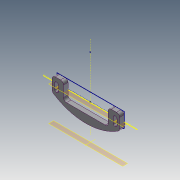
# Autodesk Inventor part: J005684
Saved by Autodesk Inventor 2015 SP1 (Build 190203100, 203)
## iProperties
Created: 2014-12-01
Material: Generic
Vendor: HHMI: JFRC - ID&F
Document SubType Name: Modeling
Designer: ARNOLDJ
Density: 1 g/cm^3
Appearance: Default
Part Number: J005684
Description: SIDE BALL GUIDE
RuleStatus: InUse
AfterDocSave0: file://Part Number Cleaner
DESIGN DEPARTMENT: HHMI: JFRC - ID&F
ALTERED ITEM PART NUMBER: N/A
ALTERED ITEM VENDOR: N/A
ALTERED ITEM DESCRIPTION: N/A
Author: ARNOLDJ
Revision Number: 0
Autodesk Inventor part; units mm, degrees
sketch "Sketch1" plane through (0, 0, 0) normal (0, 0, 1) x (1, 0, 0)
  line L0 (-100.457, 0) -> (100.457, 0) construction
  line L1 (0, 116.967) -> (0, -60.833) construction
  circle A0 centre (-62.4459, 0) radius 3.8354 construction
  circle A1 centre (62.4459, 0) radius 3.8354 construction
  line L2 (-62.4459, 0) -> (62.4459, 0) construction
  line L3 (-71.755, 17.78) -> (71.755, 17.78)
  line L4 (71.755, 17.78) -> (71.755, -13.2195)
  line L5 (-71.755, -13.2195) -> (-71.755, 17.78)
  circle A2 centre (-64.3509, 0) radius 3.8354 construction
  circle A3 centre (-60.5409, 0) radius 3.8354 construction
  line L6 (-64.3559, 3.8354) -> (-60.5409, 3.8354) construction
  line L7 (-64.3763, -3.8353) -> (-60.541, -3.8354) construction
  circle A4 centre (62.4459, 0) radius 3.8354 construction
  arc A5 (-71.755, -13.2195) -> (71.755, -13.2195) centre (0, 91.567) ccw
  line L8 (66.2813, -9.525) -> (58.6105, -9.525)
  line L9 (58.6105, -9.525) -> (58.6105, 9.525)
  line L10 (58.6105, 9.525) -> (66.2813, 9.525)
  line L11 (66.2813, 9.525) -> (66.2813, -9.525)
  line L12 (66.2813, -9.525) -> (58.6105, 9.525) construction
  line L13 (58.6105, -9.525) -> (66.2813, 9.525) construction
  line L14 (-58.6105, -9.525) -> (-66.2813, -9.525)
  line L15 (-66.2813, -9.525) -> (-66.2813, 9.525)
  line L16 (-66.2813, 9.525) -> (-58.6105, 9.525)
  line L17 (-58.6105, 9.525) -> (-58.6105, -9.525)
  line L18 (-58.6105, -9.525) -> (-66.2813, 9.525) construction
  line L19 (-66.2813, -9.525) -> (-58.6105, 9.525) construction
  point P0 (0, 0)
  point P1 (0, 0)
  point P2 (0, 17.78)
  dimension "d0" = 7.6708
  dimension "d1" = 124.8918
  dimension "d2" = 143.51
  dimension "d3" = 17.78
  dimension "d16" = 7.6708
  dimension "d17" = 1.905
  dimension "d18" = 1.905
  dimension "d33" = 127
  dimension "d34" = 19.05
  dimension "d35" = 19.05
  dimension "d36" = 7.6708
  dimension "d37" = 35.433
  constraints: 36 end point, 6 centre point, 6 midpoint, 6 point on circle, 5 coincident, 5 parallel, 4 equal radius, 4 horizontal, 4 point on line, 3 perpendicular, 2 tangent, 1 horizontal alignment, 1 vertical alignment
  measures "d0" diameter of A0
  measures "d1" distance of L2.end L2.start
  measures "d2" distance of L3.start L3.end
  measures "d3" distance from line of L3 point (0, 0)
  measures "d16" diameter of A1
  measures "d17" distance of L2.start A2.centre
  measures "d18" distance of L2.start A3.centre
  measures "d33" radius of A5
  measures "d34" distance of L10.end L8.start
  measures "d35" distance of L16.end L14.start
  measures "d36" distance of L15.end L16.end
  measures "d37" distance edge to line of A5 L2
ref_plane "Work Plane1" through (0, -74.9046, 0) normal (0, 1, 0) x (-1, 0, 0)
ref_plane "Work Plane2" through (0, -1.905, 0) normal (0, 1, 0) x (-1, 0, 0)
extrude "Extrusion1" add sketch "Sketch1" along normal blind 9.525 contours L3 L4 A5 L5 | L8 L9 L10 L11 | L14 L15 L16 L17
extrude "Extrusion3" cut sketch "Sketch1" along normal blind 9.525 contours L8 L9 L10 L11 | L14 L15 L16 L17
sketch "Sketch4" plane through (0, 0, 0) normal (0, 0, 1) x (1, 0, 0)
  line L0 (-71.755, 17.78) -> (71.755, 17.78) projected
  line L1 (-47.625, 17.78) -> (47.625, 17.78)
  line L2 (47.625, 17.78) -> (47.625, -17.78)
  line L3 (47.625, -17.78) -> (-47.625, -17.78)
  line L4 (-47.625, -17.78) -> (-47.625, 17.78)
  line L5 (0, -17.78) -> (0, 17.78) construction
  point P0 (0, 0)
  dimension "d21" = 35.56
  dimension "d22" = 95.25
  dimension "d23" = 0
  constraints: 10 end point, 2 midpoint, 2 parallel, 1 horizontal, 1 perpendicular, 1 point on line
  measures "d21" distance of L3.end L1.start
  measures "d22" distance of L2.end L3.end
  measures "d23" horizontal distance of L5.start point (0, 0)
extrude "Extrusion4" cut sketch "Sketch4" along normal up to next
fillet "Fillet2" radius 6.35 8 edges at (-47.625, -17.78, 4.7625) (-47.625, 17.78, 4.7625) (-71.755, 17.78, 4.7625) (47.625, -17.78, 4.7625) (47.625, 17.78, 4.7625) (71.755, 17.78, 4.7625) (71.755, -13.2195, 4.7625) (-71.755, -13.2195, 4.7625)
fillet "Fillet4" radius 3.175 8 edges at (-66.2813, 9.525, 4.7625) (-58.6105, 9.525, 4.7625) (-58.6105, -9.525, 4.7625) (-66.2813, -9.525, 4.7625) (58.6105, 9.525, 4.7625) (66.2813, 9.525, 4.7625) (66.2813, -9.525, 4.7625) (58.6105, -9.525, 4.7625)
sketch "Sketch5" plane through (0, 0, 0) normal (0, 0, 1) x (1, 0, 0)
  line L0 (-100.457, -1.905) -> (100.457, -1.905) projected
  line L1 (-62.4459, 0) -> (-62.4459, -1.905)
  line L2 (62.4459, 0) -> (62.4459, -1.905)
  point P0 (0, 0)
  constraints: 4 end point, 2 coincident, 2 perpendicular, 2 point on line
body "Solid1"
